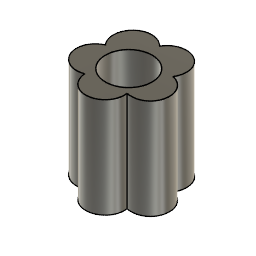
pen holder (Autodesk Fusion 360 design; units mm, degrees)
part number: 2026-07-14-22-45-19-364
Autodesk Fusion 360 part; units mm, degrees
sketch "Sketch1" plane through (0, 0, 0) normal (0, 0, 1) x (1, 0, 0)
sketch "Sketch2" plane through (0, 0, 0) normal (0, 0, 1) x (1, 0, 0)
  spline S0 degree 4 poles (-37.1693, 44.8929, 2.0524) (-49.827, 67.9335, 2.0524) (-85.2233, 67.6007, 2.0524) (-100.346, 38.962, 2.0524) (-86.7187, 15.2963, 2.0524) knots 0.11903345 0.11903345 0.11903345 0.11903345 0.11903345 0.90124376 0.90124376 0.90124376 0.90124376 0.90124376
  line L0 (-37.1693, 44.8929, 2.0524) -> (-49.827, 67.9335, 2.0524) construction
  line L1 (-49.827, 67.9335, 2.0524) -> (-85.2233, 67.6007, 2.0524) construction
  line L2 (-85.2233, 67.6007, 2.0524) -> (-100.346, 38.962, 2.0524) construction
  line L3 (-100.346, 38.962, 2.0524) -> (-86.7187, 15.2963, 2.0524) construction
  spline S1 degree 4 poles (5.2991, 5.9786, 2.0524) (22.0769, 25.1322, 2.0524) (10.9529, 56.8319, 2.0524) (-18.9169, 62.817, 2.0524) (-37.1693, 44.8929, 2.0524) knots 0.11903345 0.11903345 0.11903345 0.11903345 0.11903345 0.87667324 0.87667324 0.87667324 0.87667324 0.87667324
  line L4 (5.2991, 5.9786, 2.0524) -> (22.0769, 25.1322, 2.0524) construction
  line L5 (22.0769, 25.1322, 2.0524) -> (10.9529, 56.8319, 2.0524) construction
  line L6 (10.9529, 56.8319, 2.0524) -> (-18.9169, 62.817, 2.0524) construction
  line L7 (-18.9169, 62.817, 2.0524) -> (-37.1693, 44.8929, 2.0524) construction
  spline S2 degree 4 poles (-16.7433, -47.2381, 2.0524) (6.9935, -56.4531, 2.0524) (32.9769, -35.158, 2.0524) (28.3849, -5.0425, 2.0524) (5.2991, 5.9786, 2.0524) knots 0.11903345 0.11903345 0.11903345 0.11903345 0.11903345 0.87667324 0.87667324 0.87667324 0.87667324 0.87667324
  line L8 (-16.7433, -47.2381, 2.0524) -> (6.9935, -56.4531, 2.0524) construction
  line L9 (6.9935, -56.4531, 2.0524) -> (32.9769, -35.158, 2.0524) construction
  line L10 (32.9769, -35.158, 2.0524) -> (28.3849, -5.0425, 2.0524) construction
  line L11 (28.3849, -5.0425, 2.0524) -> (5.2991, 5.9786, 2.0524) construction
  spline S3 degree 4 poles (-73.9661, -40.9267, 2.0524) (-78.0196, -68.1676, 2.0524) (-47.9272, -88.3743, 2.0524) (-19.2943, -73.6355, 2.0524) (-16.7433, -47.2381, 2.0524) knots 0.09122943 0.09122943 0.09122943 0.09122943 0.09122943 0.87667324 0.87667324 0.87667324 0.87667324 0.87667324
  line L12 (-73.9661, -40.9267, 2.0524) -> (-78.0196, -68.1676, 2.0524) construction
  line L13 (-78.0196, -68.1676, 2.0524) -> (-47.9272, -88.3743, 2.0524) construction
  line L14 (-47.9272, -88.3743, 2.0524) -> (-19.2943, -73.6355, 2.0524) construction
  line L15 (-19.2943, -73.6355, 2.0524) -> (-16.7433, -47.2381, 2.0524) construction
  spline S4 degree 4 poles (-86.7187, 15.2963, 2.0524) (-112.6303, 10.0184, 2.0524) (-122.4235, -23.7935, 2.0524) (-100.0123, -46.4016, 2.0524) (-73.9661, -40.9267, 2.0524) knots 0.11032757 0.11032757 0.11032757 0.11032757 0.11032757 0.88740085 0.88740085 0.88740085 0.88740085 0.88740085
  line L16 (-86.7187, 15.2963, 2.0524) -> (-112.6303, 10.0184, 2.0524) construction
  line L17 (-112.6303, 10.0184, 2.0524) -> (-122.4235, -23.7935, 2.0524) construction
  line L18 (-122.4235, -23.7935, 2.0524) -> (-100.0123, -46.4016, 2.0524) construction
  line L19 (-100.0123, -46.4016, 2.0524) -> (-73.9661, -40.9267, 2.0524) construction
  circle A0 through (-8.1136, -7.4617, -54.9375) (-60.6136, 22.8492, -54.9375) (-60.6136, -37.7726, -54.9375)
  dimension "d24" = 70
extrude "Extrude11" add sketch "Sketch2" along normal blind 150 contours S0 S1 S2 S3 S4 in plane through (0, 0, 2.0524) normal (0, 0, 1)
extrude "Extrude12" cut sketch "Sketch2" along normal blind 200 contours A0 in plane through (0, 0, -54.9375) normal (0, 0, 1)
move_body "Move1" bodies 1 to x (-1, 0, 0) y (0, 1, 0) z (0, 0, -1) at (-33.4866, 0, 304.1047)
move_body "Move2" bodies 1 to x (1, 0, 0) y (0, 1, 0) z (0, 0, 1) at (0, 0, -160)
